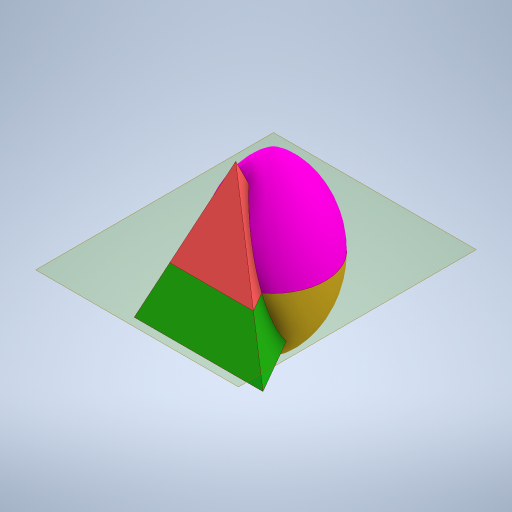
# Autodesk Inventor part: Деталька 1
Saved by Autodesk Inventor 2024 (Build 280153000, 153)
## iProperties
Created: 2023-11-09
Part Number: Деталька 1
Material: Generic
Document SubType Name: Modeling
Designer: 37525
Density: 1 g/cm^3
Appearance: Светло-красный
Author: 37525
Autodesk Inventor part; units mm, degrees
ref_plane "YZ Plane" through (0, 0, 0) normal (1, 0, 0) x (0, 1, 0)
ref_plane "XY Plane" through (0, 0, 0) normal (0, 0, 1) x (1, 0, 0)
sketch "Sketch1" plane through (0, 0, 0) normal (0, 1, 0) x (-1, 0, 0)
  circle A0 centre (-3.175, 9.525) radius 1270
  line L0 (1096.6773, 644.525) -> (-1103.0273, 644.525)
  line L1 (-1103.0273, 644.525) -> (-3.175, -1260.475)
  line L2 (-3.175, -1260.475) -> (1096.6773, 644.525)
  point P0 (0, 0)
  constraints: 6 end point, 3 point on circle, 1 centre point, 1 horizontal
ref_plane "Work Plane1" through (0, 2540, 0) normal (0, 1, 0) x (-1, 0, 0)
sketch "Sketch2" plane through (0, 2540, 0) normal (0, 1, 0) x (-1, 0, 0)
  point P0 (0, 0)
  point P1 (-3.175, 9.525)
loft "Loft1" add profiles "Sketch1" section 2 point at (3.175, 2540, 9.525) contours L2 L1 L0
sketch "Sketch3" plane through (0, 0, 0) normal (1, 0, 0) x (0, 1, 0)
  line L0 (889, -635) -> (889, -1888.649)
  line L1 (0, 644.525) -> (0, -1260.475) projected
  line L2 (889, -635) -> (1928.8125, -635)
  line L3 (1928.8125, -635) -> (-149.225, -635)
  line L4 (889, -635) -> (889, 254)
  arc A0 (2428.7932, -635) -> (-650.7932, -635) centre (889, -1524) ccw
  line L5 (2428.7932, -635) -> (-650.7932, -635)
  point P0 (0, 0)
  point P1 (-650.7932, -635)
  point P2 (-149.225, -635)
  constraints: 10 end point, 2 point on circle, 2 point on line, 1 centre point, 1 horizontal, 1 parallel, 1 vertical
revolve "Revolution1" add sketch "Sketch3" angle 360 about axis through (0, 2428.7932, -635) along (0, -1, 0)
sketch "Sketch4" plane through (1103.0273, 0, 644.525) normal (0.8401681, 0.2425356, -0.4850713) x (-0.3796283, -0.3757346, -0.8454028)
  point P0 (963.6236, 571.3208)
ref_plane "РабПлоскость3" through (0, 889, -635) normal (0, -1, 0) x (1, 0, 0)
split_face "Разделение1"
body "Solid1"
